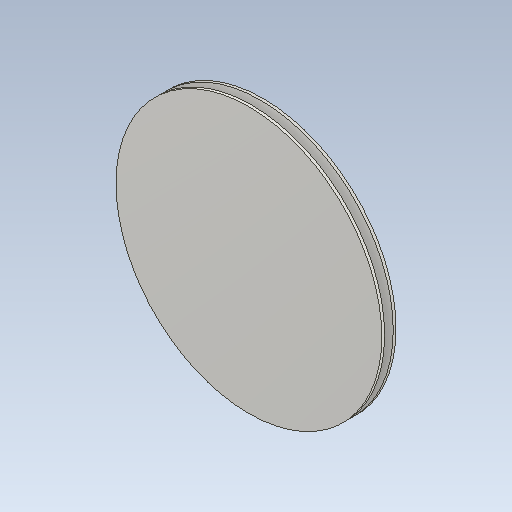
# Autodesk Inventor part: Polea ranurada2
Saved by Autodesk Inventor 2020.5 (Build 245400000, 400)
## iProperties
CustomPartVersion: 1
Created: 2022-12-03
Part Number: Polea ranurada2
Material: Steel
Document SubType Name: Modeling
Designer: André Aguirre Apolo
Density: 7.85 g/cm^3
Appearance: Steel
Author: André Aguirre Apolo
Autodesk Inventor part; units mm, degrees
ref_plane "YZ Plane" through (0, 0, 0) normal (1, 0, 0) x (0, 1, 0)
ref_plane "XZ Plane" through (0, 0, 0) normal (0, 1, 0) x (-1, 0, 0)
sketch "Boceto principal" plane through (0, 0, 0) normal (1, 0, 0) x (0, 1, 0)
  line L0 (0, 16) -> (149.5, 16)
  line L1 (149.5, 16) -> (149.5, 12.8615)
  line L2 (149.5, 12.8615) -> (138.5, 9.4984)
  line L3 (138.5, 9.4984) -> (138.5, 6.5016)
  line L4 (138.5, 6.5016) -> (149.5, 3.1385)
  line L5 (149.5, 3.1385) -> (149.5, 0)
  line L6 (149.5, 0) -> (0, 0)
  line L7 (147.5, 12.25) -> (147.5, 3.75) construction
  line L8 (138.5, 8) -> (147.5, 8) construction
  line L9 (149.5, 12.8615) -> (149.5, 3.1385)
  line L10 (0, -10.6704) -> (0, 48.4451) projected
  line L11 (0, 0) -> (0, 16)
  dimension "d0" = 8.5
  dimension "d1" = 34
  dimension "d2" = 2
  dimension "d6" = 16
  dimension "d21" = 295
  dimension "d25" = 11
  dimension "d27" = 8
  constraints: 22 end point, 5 perpendicular, 2 collinear, 2 midpoint, 2 point on line, 1 parallel
  measures "d0" distance of L7.start L7.end
  measures "d1" angle of L2 L4
  measures "d2" distance between parallel lines of L1 L7
  measures "d6" distance between parallel lines of L6 L0
  measures "d21" diameter of L7 L10
  measures "d25" distance between parallel lines of L3 L9
  measures "d27" distance between parallel lines of L6 L8
ref_plane "Plano de correa" through (0, 138.5, 8) normal (0, 0, 1) x (1, 0, 0)
revolve "Cuerpo" add sketch "Boceto principal" angle 360 about axis through (0, 0, -10) along (0, 0, 1)
revolve "Para ranuras" cut sketch "Boceto principal" angle 360 about axis through (0, 0, -10) along (0, 0, 1) contours L9 L4 L3 L2
fillet "Empalme externo" [suppressed]
fillet "Empalme interno" [suppressed]
pattern_of_one "Patrón para ranuras"
equation "\"d0\" = da_Bw"
equation "\"d1\" = da_Alfa"
equation "\"d2\" = da_c"
equation "\"d21\" = da_Dw"
equation "\"d25\" = da_Hd"
equation "\"d27\" = da_Se"
equation "\"da_r1\" = 0"
equation "\"da_r2\" = 0"
equation "\"d18\" = da_Sg"
equation "\"d5\" = da_Se"
equation "\"da_Bw\" = 8.5"
equation "\"da_Alfa\" = 34deg"
equation "\"da_c\" = 2"
equation "\"da_Dw\" = 295"
equation "\"da_Hd\" = 11"
equation "\"da_Se\" = 8"
equation "\"da_Sg\" = 12"
body "Solid1"
